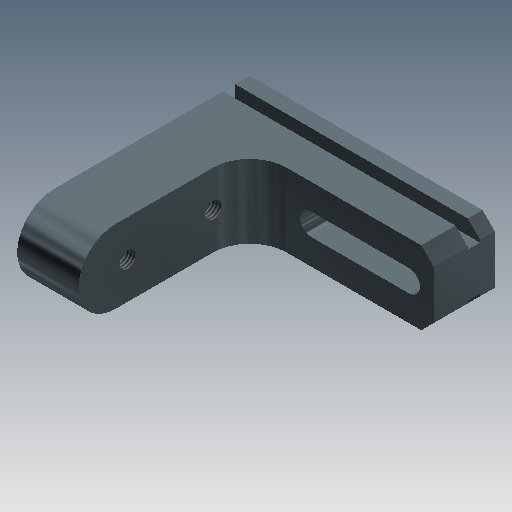
# Autodesk Inventor part: 210-102 fb
Saved by Autodesk Inventor 2020.1 (Build 241239000, 239)
## iProperties
Created: 2006-02-01
Part Number: 210-102 fb
Document SubType Name: Modeling
Designer: Kevin
Manufacturer: Standard
Standards Organization: Custom
Description: ADJUSTABLE CLAMP FINGER
Density: 1 g/cm^3
Material: Generic
Appearance: Lead
Title: BLOCK
Author: Kevin
Revision Number: -
Autodesk Inventor part; units mm, degrees
ref_plane "YZ Plane" through (0, 0, 0) normal (1, 0, 0) x (0, 1, 0)
ref_plane "XZ Plane" through (0, 0, 0) normal (0, 1, 0) x (-1, 0, 0)
sketch "Sketch2" plane through (0, 0, 0) normal (0, 0, 1) x (1, 0, 0)
  line L0 (-5.335, -2.8017) -> (69.665, -2.8017)
  line L1 (69.665, -2.8017) -> (69.665, -32.8017)
  line L2 (69.665, -32.8017) -> (-5.335, -32.8017)
  line L3 (-5.335, -32.8017) -> (-5.335, -2.8017)
  dimension "d0" = 30
  dimension "d1" = 75
  constraints: 8 end point, 2 parallel, 1 horizontal, 1 perpendicular
  measures "d0" distance of L2.end L0.start
  measures "d1" distance of L0.start L0.end
extrude "Extrusion1" add sketch "Sketch2" along normal blind 25
sketch "Sketch3" plane through (-5.335, -32.8017, 0) normal (-1, 0, 0) x (0, 0, 1)
  line L0 (25, 0) -> (25, 30) projected
  line L1 (0, 30) -> (25, 30) projected
  line L2 (0, 0) -> (0, 30) projected
  line L3 (0, 0) -> (25, 0) projected
  line L4 (25, 30) -> (80, 30)
  arc A0 (80, 0) -> (80, 30) centre (80, 15) ccw
  line L5 (80, 0) -> (25, 0)
  dimension "d15" = 80
  constraints: 4 end point, 2 parallel, 2 point on circle, 2 tangent, 1 centre point
  measures "d15" distance from line of L2 A0.centre
extrude "Extrusion2" add sketch "Sketch3" along normal blind 25
sketch "Sketch5" plane through (69.665, -32.8017, 0) normal (1, 0, 0) x (0, 0, -1)
  line L0 (0, 0) -> (-25, 0) projected
  line L1 (0, 30) -> (0, 0) projected
  line L2 (-6, 0) -> (-11, 0)
  line L3 (-11, 0) -> (-11, 6)
  line L4 (-11, 6) -> (-6, 6)
  line L5 (-6, 6) -> (-6, 0)
  dimension "d16" = 5
  dimension "d17" = 6
  dimension "d18" = 6
  constraints: 8 end point, 2 parallel, 1 horizontal, 1 perpendicular, 1 point on line
  measures "d16" distance between parallel lines of L3 L5
  measures "d17" distance between parallel lines of L2 L4
  measures "d18" distance between parallel lines of L1 L5
extrude "Extrusion4" cut sketch "Sketch5" against normal through all
ref_plane "Work Plane1" through (-5.335, -17.8017, 25) normal (0, -1, 0) x (1, 0, 0)
mirror "Mirror1" about plane through (-5.335, -17.8017, 25) normal (0, -1, 0) of "Extrusion4"
fillet "Fillet1" radius 15 1 edges at (-5.335, -17.8017, 25)
sketch "Sketch4" plane through (0, 0, 25) normal (0, 0, 1) x (1, 0, 0)
  line L0 (19.665, -13.3017) -> (59.665, -13.3017)
  arc A0 (59.665, -22.3017) -> (59.665, -13.3017) centre (59.665, -17.8017) ccw
  line L1 (59.665, -22.3017) -> (19.665, -22.3017)
  arc A1 (19.665, -13.3017) -> (19.665, -22.3017) centre (19.665, -17.8017) ccw
  line L2 (-30.335, -32.8017) -> (-30.335, -2.8017) projected
  line L3 (69.665, -32.8017) -> (9.665, -32.8017) projected
  line L4 (69.665, -2.8017) -> (69.665, -32.8017) projected
  dimension "d10" = 4.5
  dimension "d12" = 50
  dimension "d21" = 15
  dimension "d22" = 10
  constraints: 4 end point, 4 point on circle, 4 tangent, 2 centre point, 1 parallel
  measures "d10" radius of A0
  measures "d12" distance from line of L2 A1.centre
  measures "d21" distance from line of L3 A0.centre
  measures "d22" distance from line of L4 A0.centre
extrude "Extrusion3" cut sketch "Sketch4" against normal through all
chamfer "Chamfer2" distance 5 angle 45 4 edges at (69.665, -2.8017, 18) (69.665, -32.8017, 18) (69.665, -2.8017, 3) (69.665, -32.8017, 3)
sketch "Sketch9" plane through (-30.335, -32.8017, 0) normal (-1, 0, 0) x (0, 0, 1)
  line L0 (0, 0) -> (0, 30) projected
  line L1 (80, 0) -> (11, 0) projected
  point P0 (75, 15)
  point P1 (40, 15)
  dimension "d50" = 15
  dimension "d51" = 75
  dimension "d52" = 40
  constraints: 1 horizontal alignment
  measures "d50" distance from line of L1 point (75, 15)
  measures "d51" distance from line of L0 point (75, 15)
  measures "d52" distance from line of L0 point (40, 15)
hole "Hole4" at (-30.335, -17.8017, 75) at (-30.335, -17.8017, 40) direction (1, 0, 0) diameter 6.647 end through all thread size "M8x1.25" class "6H" standard "ISO Metric profile"
equation "\"d21\" = 0.5 * d0"
equation "\"d50\" = 0.5 * d0"
body "Solid1"
